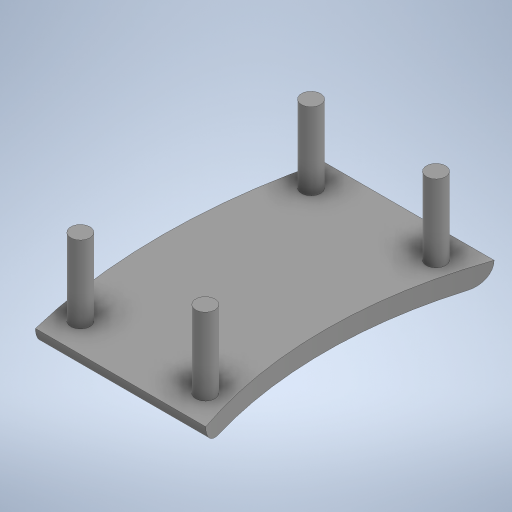
# Autodesk Inventor part: Battery Cage Spring Plate Second Iteration
Saved by Autodesk Inventor 2023 (Build 270158000, 158)
## iProperties
Created: 2023-02-15
Part Number: Battery Cage Spring Plate Second Iteration
Material: PLA 33 Plastic
Document SubType Name: Modeling
Designer: mihal
Density: 0.4135 g/cm^3
Appearance: Generic
Author: mihal
Autodesk Inventor part; units mm, degrees
ref_plane "YZ Plane" through (0, 0, 0) normal (1, 0, 0) x (0, 1, 0)
ref_plane "XZ Plane" through (0, 0, 0) normal (0, 1, 0) x (-1, 0, 0)
ref_plane "XY Plane" through (0, 0, 0) normal (0, 0, 1) x (1, 0, 0)
sketch "Sketch1" plane through (0, 0, 0) normal (0, 1, 0) x (-1, 0, 0)
  circle A0 centre (0, -75) radius 227.5
  circle A1 centre (0, -75) radius 312.5
  line L0 (214.7819, -150) -> (303.3665, -150)
  line L1 (214.7819, 0) -> (303.3665, 0)
  line L2 (437.5, 0) -> (-437.5, 0) projected
  line L3 (259.0742, 0) -> (259.0742, -150) construction
  line L4 (0, 0) -> (0, -75)
  dimension "d0" = 455
  dimension "d1" = 625
  dimension "d4" = 150
  dimension "d5" = 75
  constraints: 8 end point, 4 point on circle, 3 midpoint, 2 centre point, 2 parallel, 1 coincident, 1 perpendicular, 1 point on line, 1 vertical
  measures "d0" diameter of A0
  measures "d1" diameter of A1
  measures "d4" distance of L3.start L3.end
  measures "d5" distance of L4.start L4.end
extrude "Extrusion1" add sketch "Sketch1" along normal blind 10 contours A0 L1 A1 L0
sketch "Sketch2" plane through (0, 10, 0) normal (0, 1, 0) x (1, 0, 0)
  arc A0 (-214.7819, 150) -> (-214.7819, 0) centre (0, 75) ccw projected
  line L0 (-214.7819, 150) -> (-303.3665, 150) projected
  arc A1 (-303.3665, 150) -> (-303.3665, 0) centre (0, 75) ccw projected
  line L1 (-303.3665, 0) -> (-214.7819, 0) projected
  line L2 (-227.5, 75) -> (-312.5, 75) construction
  line L3 (-270, 75) -> (-270, 150) construction
  line L4 (-270, 75) -> (-270, 0) construction
  line L5 (-295, 25) -> (-245, 25)
  line L6 (-245, 25) -> (-245, 125)
  line L7 (-245, 125) -> (-295, 125)
  line L8 (-295, 125) -> (-295, 25)
  line L9 (-295, 75) -> (-245, 75) construction
  line L10 (-270, 25) -> (-270, 125) construction
  line L11 (-295, 25) -> (-295, 15) construction
  line L12 (-245, 25) -> (-245, 15) construction
  line L13 (-245, 25) -> (-235, 25) construction
  line L14 (-245, 15) -> (-230, 15) construction
  line L15 (-245, 125) -> (-245, 135) construction
  line L16 (-245, 135) -> (-230, 135) construction
  line L17 (-295, 125) -> (-295, 135) construction
  circle A2 centre (-295, 15) radius 5
  circle A3 centre (-230, 15) radius 5
  circle A4 centre (-230, 135) radius 5
  circle A5 centre (-295, 135) radius 5
  point P0 (0, 0)
  dimension "d8" = 50
  dimension "d9" = 100
  dimension "d10" = 10
  dimension "d11" = 10
  dimension "d12" = 90
  dimension "d13" = 15
  dimension "d14" = 10
  dimension "d15" = 15
  dimension "d16" = 90
  dimension "d17" = 10
  dimension "d18" = 10
  dimension "d19" = 10
  dimension "d20" = 10
  dimension "d21" = 10
  constraints: 32 end point, 6 midpoint, 5 perpendicular, 4 centre point, 4 coincident, 4 vertical, 3 point on line, 2 horizontal, 2 parallel, 2 point on circle
  measures "d8" distance of L7.end L6.end
  measures "d9" distance of L6.end L5.end
  measures "d10" distance of L5.start L11.end
  measures "d11" distance of L5.end L12.end
  measures "d12" angle of L12 L13
  measures "d13" distance of L12.end L14.end
  measures "d14" distance of L6.end L15.end
  measures "d15" distance of L15.end L16.end
  measures "d16" angle of L15 L16
  measures "d17" distance of L7.end L17.end
  measures "d18" diameter of A2
  measures "d19" diameter of A3
  measures "d20" diameter of A4
  measures "d21" diameter of A5
extrude "Extrusion2" add sketch "Sketch2" along normal blind 40 contours A2 | A3 | A4 | A5
fillet "Fillet1" radius 10 2 edges at (-259.0742, 0, 0) (-259.0742, 0, -150)
body "Solid1"
